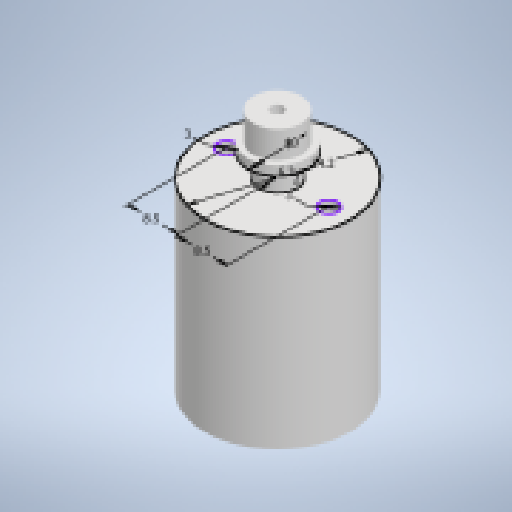
# Autodesk Inventor part: Motor
Saved by Autodesk Inventor 2023.1 (Build 271208000, 208)
## iProperties
Created: 2024-02-14
Part Number: Motor
Material: Generic
Document SubType Name: Modeling
Designer: USER
Density: 1 g/cm^3
Appearance: Default
Author: USER
Autodesk Inventor part; units mm, degrees
ref_plane "YZ Plane" through (0, 0, 0) normal (1, 0, 0) x (0, 1, 0)
ref_plane "XZ Plane" through (0, 0, 0) normal (0, 1, 0) x (-1, 0, 0)
ref_plane "XY Plane" through (0, 0, 0) normal (0, 0, 1) x (1, 0, 0)
sketch "Sketch1" plane through (0, 0, 0) normal (0, 1, 0) x (-1, 0, 0)
  circle A0 centre (0, 0) radius 12.1
  circle A1 centre (0, 0) radius 3.15
  circle A2 centre (0, 0) radius 1
  circle A3 centre (-8.5, 0) radius 1.5
  circle A4 centre (8.5, 0) radius 1.5
  dimension "d0" = 24.2
  dimension "d1" = 6.3
  dimension "d6" = 2
  dimension "d16" = 3
  dimension "d17" = 3
  dimension "d18" = 8.5
  dimension "d19" = 8.5
  constraints: 5 centre point, 3 coincident
  measures "d0" diameter of A0
  measures "d1" diameter of A1
  measures "d6" diameter of A2
  measures "d16" diameter of A3
  measures "d17" diameter of A4
  measures "d18" distance of point (0, 0) A3.centre
  measures "d19" distance of A4.centre point (0, 0)
extrude "Extrusion1" add sketch "Sketch1" against normal blind 30.7 contours A0 | A1 | A2 | A3 | A4
extrude "Extrusion2" add sketch "Sketch1" along normal blind 2 contours A1 | A2
extrude "Extrusion3" add sketch "Sketch1" along normal blind 8.5 contours A2
ref_plane "Work Plane1" through (0, 3.7375, 0) normal (0, 1, 0) x (1, 0, 0)
sketch "Sketch2" plane through (0, 3.7375, 0) normal (0, 1, 0) x (1, 0, 0)
  circle A0 centre (0, 0) radius 5
  circle A1 centre (0, 0) radius 1 projected
  circle A2 centre (0, 0) radius 4
  dimension "d10" = 10
  dimension "d11" = 8
  constraints: 2 centre point, 2 coincident
  measures "d10" diameter of A0
  measures "d11" diameter of A2
extrude "Extrusion4" add sketch "Sketch2" along normal blind 1.5 contours A0 | A2
extrude "Extrusion5" add sketch "Sketch2" along normal blind 6 contours A2
extrude "Extrusion6" cut sketch "Sketch1" against normal blind 5 contours A3 | A4
body "Solid1"
